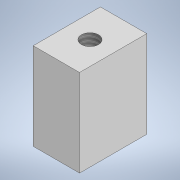
# Autodesk Inventor part: test1
Saved by Autodesk Inventor 2020.3 (Build 243373000, 373)
## iProperties
Created: 2020-05-27
Part Number: test1
Material: Generic
Document SubType Name: Modeling
Designer: robst
Density: 1 g/cm^3
Appearance: Default
Author: robst
Autodesk Inventor part; units mm, degrees
ref_plane "YZ Plane" through (0, 0, 0) normal (1, 0, 0) x (0, 1, 0)
ref_plane "XZ Plane" through (0, 0, 0) normal (0, 1, 0) x (-1, 0, 0)
ref_plane "XY Plane" through (0, 0, 0) normal (0, 0, 1) x (1, 0, 0)
sketch "Sketch1" plane through (0, 0, 0) normal (0, 1, 0) x (-1, 0, 0)
  line L0 (-6.751, 9.7956) -> (-6.751, -9.7956)
  line L1 (-6.751, -9.7956) -> (6.751, -9.7956)
  line L2 (6.751, -9.7956) -> (6.751, 9.7956)
  line L3 (6.751, 9.7956) -> (-6.751, 9.7956)
  line L4 (-6.751, 9.7956) -> (6.751, -9.7956) construction
  line L5 (-6.751, -9.7956) -> (6.751, 9.7956) construction
  point P0 (0, 0)
  constraints: 12 end point, 2 midpoint, 2 parallel, 1 perpendicular, 1 vertical
extrude "Extrusion1" add sketch "Sketch1" against normal blind 25.4
sketch "Sketch2" plane through (0, 0, 0) normal (0, 1, 0) x (1, 0, 0)
  point P0 (0, 0)
  point P1 (0, 0)
  constraints: 1 coincident
hole "Hole1" at (0, 0, 0) direction (0, -1, 0) diameter 4.9784 end through all thread size "1/4-20 UNC" class "2B" standard "ANSI Unified Screw Threads"
body "Solid1"
